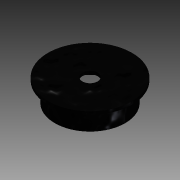
# Autodesk Inventor part: Plastic Lid
Saved by Autodesk Inventor 2014 (Build 180170000, 170)
## iProperties
Created: 2014-06-10
Part Number: Plastic Lid
Material: Generic
Document SubType Name: Modeling
Designer: Nabeel
Density: 1 g/cm^3
Appearance: Default
Author: Nabeel
Autodesk Inventor part; units mm, degrees
ref_plane "YZ Plane" through (0, 0, 0) normal (1, 0, 0) x (0, 1, 0)
ref_plane "XZ Plane" through (0, 0, 0) normal (0, 1, 0) x (-1, 0, 0)
ref_plane "XY Plane" through (0, 0, 0) normal (0, 0, 1) x (1, 0, 0)
ref_plane "Work Plane1" through (0, 0, 76.3) normal (0, 0, 1) x (1, 0, 0)
ref_plane "Work Plane2" through (0, 0, 89) normal (0, 0, 1) x (1, 0, 0)
sketch "Sketch4" plane through (0, 0, 89) normal (0, 0, 1) x (1, 0, 0)
  circle A0 centre (0, 0) radius 23.5 projected
  circle A1 centre (0, 0) radius 23
  dimension "d20" = 46
  constraints: 1 centre point, 1 coincident
  measures "d20" diameter of A1
extrude "Extrusion4" add sketch "Sketch4" along normal blind 12.7 contours A1
sketch "Sketch5" plane through (0, 0, 101.7) normal (0, 0, 1) x (1, 0, 0)
  circle A0 centre (0, 0) radius 23 projected
  circle A1 centre (0, 0) radius 23 projected
hole "Hole2" at (0, 0, 101.7) direction (0, 0, -1) diameter 45 depth 12.8
sketch "Sketch6" plane through (0, 0, 101.7) normal (0, 0, 1) x (1, 0, 0)
  circle A0 centre (0, 0) radius 22.5 projected
  circle A1 centre (0, 0) radius 23 projected
  line L0 (0, -38.5) -> (0, 38.5) projected
  line L1 (-38.5, 0) -> (38.5, 0) projected
  circle A2 centre (0, 0) radius 27.5
  dimension "d30" = 55
  constraints: 1 centre point, 1 coincident
  measures "d30" diameter of A2
extrude "Extrusion5" add sketch "Sketch6" along normal blind 2
sketch "Sketch7" plane through (0, 0, 103.7) normal (0, 0, 1) x (1, 0, 0)
  circle A0 centre (0, 0) radius 27.5 projected
  line L0 (0, -38.5) -> (0, 38.5) projected
  line L1 (-38.5, 0) -> (38.5, 0) projected
hole "Hole3" at (0, 0, 103.7) direction (0, 0, -1) diameter 10 depth 8 tip angle 118
body "Solid1"
